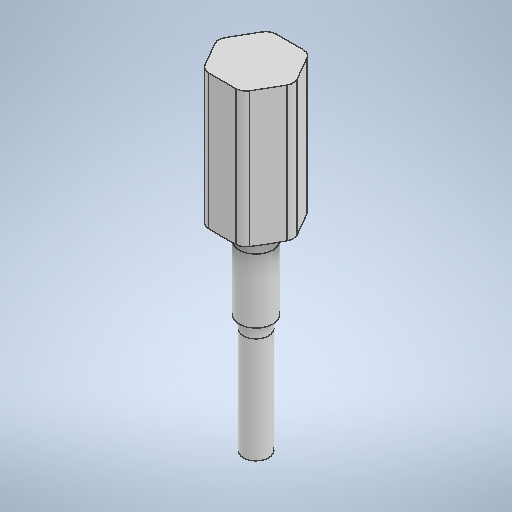
# Autodesk Inventor part: jig
Saved by Autodesk Inventor 2025 (Build 290162000, 162)
## iProperties
Created: 2026-02-28
Part Number: jig
Material: 一般
Document SubType Name: Modeling
Designer: sooo1
Density: 1 g/cm^3
Appearance: 既定
Author: sooo1
Autodesk Inventor part; units mm, degrees
ref_plane "YZ Plane" through (0, 0, 0) normal (1, 0, 0) x (0, 1, 0)
ref_plane "XZ Plane" through (0, 0, 0) normal (0, 1, 0) x (-1, 0, 0)
sketch "スケッチ1" plane through (0, 0, 0) normal (0, 1, 0) x (-1, 0, 0)
  circle A0 centre (0, 0) radius 3.75
  line L0 (-2.8868, 0) -> (-1.4434, 2.5) construction
  line L1 (-1.4434, 2.5) -> (1.4434, 2.5) construction
  line L2 (1.4434, 2.5) -> (2.8868, 0) construction
  line L3 (2.8868, 0) -> (1.4434, -2.5) construction
  line L4 (1.4434, -2.5) -> (-1.4434, -2.5) construction
  line L5 (-1.4434, -2.5) -> (-2.8868, 0) construction
  line L6 (16.1658, 0) -> (-16.1658, 0) construction
  line L7 (3.0022, 0) -> (1.5011, 2.6)
  line L8 (1.5011, 2.6) -> (-1.5011, 2.6)
  line L9 (-1.5011, 2.6) -> (-3.0022, 0)
  line L10 (-3.0022, 0) -> (-1.5011, -2.6)
  line L11 (-1.5011, -2.6) -> (1.5011, -2.6)
  line L12 (1.5011, -2.6) -> (3.0022, 0)
  circle A1 centre (0, 0) radius 1.5
  circle A2 centre (0, 0) radius 5
  line L13 (-1.1, 1.6) -> (1.1, 1.6)
  line L14 (1.1, 1.6) -> (1.1, -1.6)
  line L15 (1.1, -1.6) -> (-1.1, -1.6)
  line L16 (-1.1, -1.6) -> (-1.1, 1.6)
  line L17 (-1.1, 1.6) -> (1.1, -1.6) construction
  line L18 (1.1, 1.6) -> (-1.1, -1.6) construction
  line L19 (11.547, 0) -> (5.7735, -10)
  line L20 (5.7735, -10) -> (-5.7735, -10)
  line L21 (-5.7735, -10) -> (-11.547, 0)
  line L22 (-11.547, 0) -> (-5.7735, 10)
  line L23 (-5.7735, 10) -> (5.7735, 10)
  line L24 (5.7735, 10) -> (11.547, 0)
  line L25 (1.5011, 2.6) -> (4.2708, 2.6)
  line L26 (1.5011, -2.6) -> (4.2708, -2.6)
  point P0 (0, 0)
  dimension "d0" = 5
  dimension "d1" = 0.1
  dimension "d2" = 7.5
  dimension "d7" = 3
  dimension "d10" = 10
  dimension "d16" = 2.2
  dimension "d17" = 3.2
  dimension "d25" = 20
  constraints: 52 end point, 4 coincident, 3 centre point, 3 parallel, 2 horizontal, 2 midpoint, 2 point on circle, 2 point on line, 1 perpendicular, 31 other
  measures "d0" distance between parallel lines of L0 L3
  measures "d1" distance between parallel lines of L3 L12
  measures "d2" diameter of A0
  measures "d7" diameter of A1
  measures "d10" diameter of A2
  measures "d16" distance of L13.start L13.end
  measures "d17" distance of L15.end L13.start
  measures "d25" distance between parallel lines of L23 L20
extrude "押し出し1" add sketch "スケッチ1" along normal blind 7.5 contours A0 L26 L12 L7 L25 | L25 L8 L9 L10 L11 L26 A0 | L7 L12 L11 L10 L9 L8 | A1 L14 | L14 A1 L16 | A1 L16 L13 L14 | L14 L15 L16 A1 | L16 A1
extrude "押し出し2" cut sketch "スケッチ1" along normal blind 2 contours L7 L12 L11 L10 L9 L8 | A1 L14 | L14 A1 L16 | A1 L16 L13 L14 | L14 L15 L16 A1 | L16 A1
ref_plane "作業平面1" through (0, 3, 0) normal (0, -1, 0) x (1, 0, 0)
extrude "押し出し3" cut sketch "スケッチ1" along normal through all contours A1 L14 | L14 A1 L16 | L16 A1
extrude "押し出し6" cut sketch "スケッチ1" along normal blind 3.5 from surface at 3 contours L14 A1 L16 | A1 L16 L13 L14 | L14 L15 L16 A1
extrude "押し出し7" add sketch "スケッチ1" along normal blind 27.5 from surface at 7.5 contours A0 L26 L12 L7 L25 | L25 L8 L9 L10 L11 L26 A0 | L7 L12 L11 L10 L9 L8 | A1 L14 | L14 A1 L16 | A1 L16 L13 L14 | L14 L15 L16 A1 | L16 A1
extrude "押し出し8" add sketch "スケッチ1" along normal blind 25 from surface at 35 contours A0 L26 L12 L7 L25 | A0 L25 A2 L26 | L25 L8 L9 L10 L11 L26 A0 | A0 L26 A2 L25 | L7 L12 L11 L10 L9 L8 | A1 L14 | L14 A1 L16 | A1 L16 L13 L14 | L14 L15 L16 A1 | L16 A1
extrude "押し出し9" add sketch "スケッチ1" along normal blind 40 from surface at 60 contours A0 L26 L12 L7 L25 | A0 L25 A2 L26 | L25 L8 L9 L10 L11 L26 A0 | A0 L26 A2 L25 | L7 L12 L11 L10 L9 L8 | A1 L14 | L14 A1 L16 | A1 L16 L13 L14 | L14 L15 L16 A1 | L16 A1 | L19 L20 L21 L22 L23 L24
fillet "フィレット1" radius 6 1 edges at (5, 60, 0)
fillet "フィレット2" radius 6 1 edges at (3.75, 35, 0)
fillet "フィレット3" radius 3 6 edges at (-5.7735, 80, -10) (5.7735, 80, -10) (11.547, 80, 0) (5.7735, 80, 10) (-5.7735, 80, 10) (-11.547, 80, 0)
chamfer "面取り1" distance 0.2 angle 45 6 edges at (-2.2517, 0, 1.3) (0, 0, 2.6) (-2.2517, 0, -1.3) (0, 0, -2.6) (2.2517, 0, -1.3) (2.2517, 0, 1.3)
